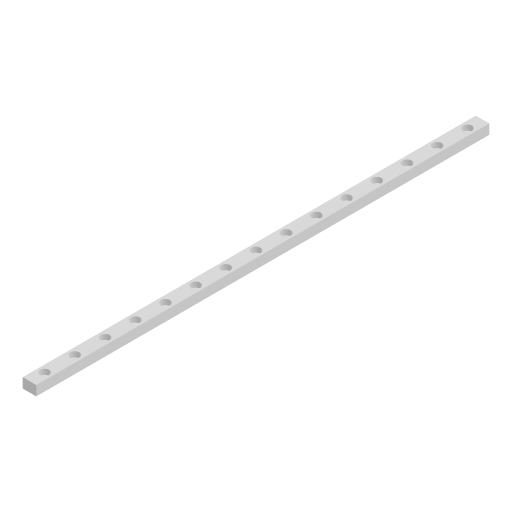
# Autodesk Inventor part: mgn9 350mm
Saved by Autodesk Inventor 2023 (Build 270158000, 158)
## iProperties
Created: 2022-09-16
Part Number: mgn9 350mm
Material: Generic
Document SubType Name: Modeling
Designer: deli
Density: 1 g/cm^3
Appearance: Default
Author: deli
Autodesk Inventor part; units mm, degrees
ref_plane "YZ Plane" through (0, 0, 0) normal (1, 0, 0) x (0, 1, 0)
ref_plane "XZ Plane" through (0, 0, 0) normal (0, 1, 0) x (-1, 0, 0)
ref_plane "XY Plane" through (0, 0, 0) normal (0, 0, 1) x (1, 0, 0)
sketch "Sketch4" plane through (0, 0, 0) normal (0, 0, 1) x (1, 0, 0)
  line L0 (-22.685, 6.9816) -> (-13.685, 6.9816)
  line L1 (-13.685, 6.9816) -> (-13.685, 0.4816)
  line L2 (-13.685, 0.4816) -> (-22.685, 0.4816)
  line L3 (-22.685, 0.4816) -> (-22.685, 6.9816)
  point P0 (0, 0)
  dimension "d27" = 9
  dimension "d28" = 6.5
  constraints: 8 end point, 2 parallel, 1 horizontal, 1 perpendicular
  measures "d27" distance of L1.end L2.end
  measures "d28" distance of L0.end L1.end
extrude "Extrusion3" add sketch "Sketch4" along normal blind 300
sketch "Sketch7" plane through (-22.685, 6.9816, 0) normal (0, 1, 0) x (1, 0, 0)
  circle A0 centre (4.5, -10) radius 1.75
  line L0 (9, 0) -> (9, -300) projected
  circle A1 centre (4.5, -30) radius 1.75
  circle A2 centre (4.5, -50) radius 1.75
  circle A3 centre (4.5, -70) radius 1.75
  circle A4 centre (4.5, -90) radius 1.75
  circle A5 centre (4.5, -110) radius 1.75
  circle A6 centre (4.5, -130) radius 1.75
  circle A7 centre (4.5, -150) radius 1.75
  circle A8 centre (4.5, -170) radius 1.75
  circle A9 centre (4.5, -190) radius 1.75
  circle A10 centre (4.5, -210) radius 1.75
  circle A11 centre (4.5, -230) radius 1.75
  circle A12 centre (4.5, -250) radius 1.75
  circle A13 centre (4.5, -270) radius 1.75
  circle A14 centre (4.5, -290) radius 1.75
  line L1 (9, 0) -> (0, 0) projected
  point P0 (22.685, 0)
  dimension "d38" = 3.5
  dimension "d39" = 4.5
  dimension "d45" = 20
  dimension "d47" = 280
  dimension "d48" = 10
  constraints: 15 centre point, 1 vertical, 28 other
  measures "d38" diameter of A0
  measures "d39" distance from line of L0 A0.centre
  measures "d45" distance of A0.centre A1.centre
  measures "d47" distance of A14.centre A0.centre
  measures "d48" distance from line of A0.centre L1
extrude "Extrusion6" cut sketch "Sketch7" against normal blind 10
sketch "Sketch8" plane through (-22.685, 6.9816, 0) normal (0, 1, 0) x (1, 0, 0)
  circle A0 centre (4.5, -10) radius 1.75 construction
  circle A1 centre (4.5, -10) radius 3
  line L0 (9, 0) -> (9, -300) projected
  line L1 (9, 0) -> (0, 0) projected
  line L2 (0, 0) -> (0, -300) projected
  line L3 (14.5, -300) -> (-5.5, -300) projected
  circle A2 centre (4.5, -30) radius 3
  circle A3 centre (4.5, -50) radius 3
  circle A4 centre (4.5, -70) radius 3
  circle A5 centre (4.5, -90) radius 3
  circle A6 centre (4.5, -110) radius 3
  circle A7 centre (4.5, -130) radius 3
  circle A8 centre (4.5, -150) radius 3
  circle A9 centre (4.5, -170) radius 3
  circle A10 centre (4.5, -190) radius 3
  circle A11 centre (4.5, -210) radius 3
  circle A12 centre (4.5, -230) radius 3
  circle A13 centre (4.5, -250) radius 3
  circle A14 centre (4.5, -270) radius 3
  circle A15 centre (4.5, -290) radius 3
  point P0 (22.685, 0)
  dimension "d51" = 6
  dimension "d57" = 20
  constraints: 15 centre point, 1 coincident, 1 vertical, 28 other
  measures "d51" diameter of A1
  measures "d57" distance of A1.centre A2.centre
extrude "Extrusion7" cut sketch "Sketch8" against normal blind 3.5 contours A1 | A2 | A3 | A4 | A5 | A6 | A7 | A8 | A9 | A10 | A11 | A12 | A13 | A14 | A15
body "Solid2"
